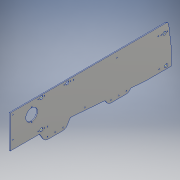
# Autodesk Inventor part: Storage Side Plate
Saved by Autodesk Inventor 2019.4 (Build 234330000, 330)
## iProperties
Created: 2020-01-24
Part Number: Storage Side Plate
Material: Aluminum 6061
Document SubType Name: Modeling
Designer: admin
Density: 2.7 g/cm^3
Appearance: Aluminum - Flat
Mass: 2534.1 g
Surface Area: 3913.12 cm^2
Volume: 938.555 cm^3
Author: admin
Autodesk Inventor part; units mm, degrees
ref_plane "YZ Plane" through (0, 0, 0) normal (1, 0, 0) x (0, 1, 0)
ref_plane "XZ Plane" through (0, 0, 0) normal (0, 1, 0) x (-1, 0, 0)
ref_plane "XY Plane" through (0, 0, 0) normal (0, 0, 1) x (1, 0, 0)
sketch "Sketch1" plane through (0, 0, 0) normal (1, 0, 0) x (0, 1, 0)
  line L0 (0, 0) -> (190, 0)
  line L1 (190, 0) -> (190, -912)
  circle A0 centre (97, -465) radius 88.9 construction
  circle A1 centre (177, -180) radius 9.5
  circle A2 centre (17, -180) radius 9.5
  circle A3 centre (-23, -898.888) radius 9.5
  circle A4 centre (143.8889, -889.1351) radius 9.5
  line L2 (17, -180) -> (-23, -898.888) construction
  line L3 (234.971, -205) -> (-89.3496, -205) construction
  circle A5 centre (175, -330) radius 9.5
  line L4 (175, -330) -> (143.8889, -889.1351) construction
  line L5 (17, -180) -> (177, -180) construction
  circle A6 centre (97, -268.8359) radius 88.9 construction
  circle A7 centre (-93.9984, -625.4651) radius 88.9 construction
  circle A8 centre (-75.5805, -1096.5117) radius 88.9 construction
  circle A9 centre (173.0556, -364.9459) radius 2.75
  circle A10 centre (159.1667, -614.5598) radius 2.75
  circle A11 centre (145.8333, -854.1892) radius 2.75
  circle A12 centre (-20.7778, -858.9498) radius 2.75
  circle A13 centre (-9.1111, -649.2741) radius 2.75
  circle A14 centre (3.1111, -429.6139) radius 2.75
  circle A15 centre (15.0556, -214.9459) radius 2.75
  circle A16 centre (50, -15) radius 2.75
  circle A17 centre (175, -15) radius 2.75
  line L6 (-40, -930) -> (40, -930)
  line L7 (40, -930) -> (190, -912)
  circle A18 centre (-10.6816, -885.7633) radius 2.5 construction
  circle A19 centre (-35.3184, -912.0127) radius 2.5 construction
  line L8 (143.8889, -871.1351) -> (143.8889, -907.1351) construction
  circle A20 centre (143.8889, -871.1351) radius 2.5
  circle A21 centre (143.8889, -907.1351) radius 2.5
  line L9 (17, -162) -> (17, -198) construction
  circle A22 centre (17, -162) radius 2.5
  circle A23 centre (17, -198) radius 2.5
  line L10 (175, -312) -> (175, -348) construction
  circle A24 centre (175, -312) radius 2.5
  circle A25 centre (175, -348) radius 2.5
  line L11 (177, -162) -> (177, -198) construction
  circle A26 centre (177, -162) radius 2.5
  circle A27 centre (177, -198) radius 2.5
  line L12 (-10.6816, -885.7633) -> (-35.3184, -912.0127) construction
  line L13 (0, 0) -> (0, -280)
  line L14 (0, -280) -> (-40, -780)
  line L15 (-40, -780) -> (-40, -930)
  dimension "d1" = 177.8
  dimension "d2" = 19
  dimension "d3" = 19
  dimension "d4" = 19
  dimension "d5" = 19
  dimension "d8" = 180
  dimension "d9" = 180
  dimension "d10" = 205
  dimension "d11" = 19
  dimension "d14" = 125
  dimension "d15" = 190
  dimension "d16" = 18
  dimension "d19" = 160
  dimension "d20" = 560
  dimension "d21" = 720
  dimension "d22" = 177.8
  dimension "d23" = 177.8
  dimension "d24" = 177.8
  dimension "d35" = 5.5
  dimension "d36" = 5.5
  dimension "d37" = 5.5
  dimension "d38" = 35
  dimension "d39" = 35
  dimension "d40" = 250
  dimension "d41" = 5.5
  dimension "d42" = 5.5
  dimension "d43" = 5.5
  dimension "d44" = 5.5
  dimension "d45" = 5.5
  dimension "d46" = 5.5
  dimension "d47" = 35
  dimension "d48" = 40
  dimension "d49" = 250
  dimension "d50" = 250
  dimension "d52" = 15
  dimension "d53" = 15
  dimension "d54" = 15
  dimension "d55" = 80
  dimension "d81" = 5
  dimension "d82" = 5
  dimension "d83" = 36
  dimension "d84" = 5
  dimension "d85" = 5
  dimension "d86" = 36
  dimension "d87" = 5
  dimension "d88" = 5
  dimension "d89" = 36
  dimension "d90" = 5
  dimension "d91" = 5
  dimension "d92" = 36
  dimension "d93" = 5
  dimension "d94" = 5
  dimension "d95" = 36
  dimension "d105" = 930
  dimension "d106" = 40
  dimension "d108" = 50
  dimension "d109" = 500
  dimension "d110" = 17
  dimension "d111" = 17
  dimension "d112" = 40
  dimension "d113" = 150
  dimension "d114" = 15
  constraints: 32 end point, 28 centre point, 10 coincident, 7 point on line, 5 midpoint, 5 vertical, 3 horizontal, 2 parallel, 1 perpendicular
  measures "d1" diameter of A0
  measures "d2" diameter of A1
  measures "d3" diameter of A2
  measures "d4" diameter of A3
  measures "d5" diameter of A4
  measures "d8" distance from line of L5.end L0
  measures "d9" distance from line of L2.start L0
  measures "d10" distance between parallel lines of L0 L3
  measures "d11" diameter of A5
  measures "d14" distance from line of L4.start L3
  measures "d15" distance of L0.start L0.end
  measures "d16" vertical distance of L1.end L6.start
  measures "d19" distance of L2.start L5.end
  measures "d20" distance of L4.end L4.start
  measures "d21" distance of L2.end L2.start
  measures "d22" diameter of A6
  measures "d23" diameter of A7
  measures "d24" diameter of A8
  measures "d35" diameter of A9
  measures "d36" diameter of A10
  measures "d37" diameter of A11
  measures "d38" distance of L4.start A9.centre
  measures "d39" distance of L4.end A11.centre
  measures "d40" distance of A9.centre A10.centre
  measures "d41" diameter of A12
  measures "d42" diameter of A13
  measures "d43" diameter of A14
  measures "d44" diameter of A15
  measures "d45" diameter of A16
  measures "d46" diameter of A17
  measures "d47" distance of L2.start A15.centre
  measures "d48" distance of L2.end A12.centre
  measures "d49" distance of L2.end A13.centre
  measures "d50" distance of L2.start A14.centre
  measures "d52" distance from line of L1 A17.centre
  measures "d53" distance from line of L0 A17.centre
  measures "d54" distance from line of L0 A16.centre
  measures "d55" distance of L6.start L6.end
  measures "d81" diameter of A18
  measures "d82" diameter of A19
  measures "d83" distance of L8.start L8.end
  measures "d84" diameter of A20
  measures "d85" diameter of A21
  measures "d86" distance of L9.start L9.end
  measures "d87" diameter of A22
  measures "d88" diameter of A23
  measures "d89" distance of L10.start L10.end
  measures "d90" diameter of A24
  measures "d91" diameter of A25
  measures "d92" distance of L11.start L11.end
  measures "d93" diameter of A26
  measures "d94" diameter of A27
  measures "d95" distance of L12.start L12.end
  measures "d105" distance between parallel lines of L0 L6
  measures "d106" horizontal distance of L13.end L14.end
  measures "d108" distance from line of L13 A16.centre
  measures "d109" vertical distance of L13.end L14.end
  measures "d110" distance from line of L13 L2.start
  measures "d111" distance from line of L15 L2.end
  measures "d112" angle of L2 L12
  measures "d113" distance of L14.end L6.start
  measures "d114" distance from line of L1 L4.start
extrude "Extrusion1" add sketch "Sketch1" along normal blind 5
ref_plane "Work Plane3" through (5, 1011.7922, 17698.6054) normal (0, -0.9986936, 0.051099) x (-1, 0, 0)
ref_plane "Work Plane1" through (5, 177, -180) normal (0, -0.9989117, 0.0466414) x (-1, 0, 0)
ref_plane "Work Plane2" through (5, -23, -898.888) normal (0, 0.9984556, -0.0555556) x (-1, 0, 0)
ref_plane "Work Plane5" through (5, 177, -245) normal (0, 0, 1) x (-1, 0, 0)
ref_plane "Work Plane4" through (5, 177, -180) normal (0, 0, 1) x (-1, 0, 0)
fillet "Fillet1" radius 15 1 edges at (2.5, 190, -912)
sketch "Sketch2" plane through (5, 0, 0) normal (1, 0, 0) x (0, 0, -1)
  line L0 (780, -40) -> (930, -40) projected
  line L1 (930, -40) -> (865, -40)
  line L2 (865, -40) -> (865, -35)
  line L3 (865, -35) -> (930, -35)
  line L4 (930, -35) -> (930, -40)
  dimension "d115" = 65
  dimension "d116" = 5
  constraints: 8 end point, 2 parallel, 1 horizontal, 1 perpendicular
  measures "d115" distance of L2.end L3.end
  measures "d116" distance of L1.end L2.end
extrude "Extrusion2" [suppressed]
fillet "Fillet3" [suppressed]
sketch "Sketch4" plane through (5, 0, 0) normal (1, 0, 0) x (0, 0, -1)
  circle A0 centre (10, 14.3) radius 2.75 projected
  circle A1 centre (400.3762, 175) radius 2.75 projected
  circle A2 centre (437.8762, 175) radius 2.75 projected
  circle A3 centre (475.3762, 175) radius 2.75 projected
  circle A4 centre (512.8762, 175) radius 2.75 projected
  circle A5 centre (550.3762, 175) radius 2.75 projected
  circle A6 centre (220.7003, 175) radius 2.75 projected
  circle A7 centre (250.7003, 175) radius 2.75 projected
  circle A8 centre (280.7003, 175) radius 2.75 projected
  circle A9 centre (882, -23) radius 2.75 projected
  circle A10 centre (918, -23) radius 2.75 projected
  point P0 (0, 0)
extrude "Extrusion4" [suppressed]
sketch "Sketch5" plane through (5, 0, 0) normal (1, 0, 0) x (0, 0, -1)
  line L0 (865, 0) -> (0, 0) projected
  line L1 (170, 0) -> (200, -50)
  line L2 (200, -50) -> (320, -50)
  line L3 (320, -50) -> (350, 0)
  line L4 (535, 0) -> (565, -50)
  line L5 (565, -50) -> (685, -50)
  line L6 (685, -50) -> (715, 0)
  line L7 (215, -35) -> (305, -35) construction
  circle A0 centre (215, -35) radius 2.75
  circle A1 centre (305, -35) radius 2.75
  circle A2 centre (260, -35) radius 2.75
  line L8 (260, -35) -> (260, -50) construction
  line L9 (580, -35) -> (670, -35) construction
  circle A3 centre (580, -35) radius 2.75
  circle A4 centre (670, -35) radius 2.75
  circle A5 centre (625, -35) radius 2.75
  line L10 (625, -35) -> (625, -50) construction
  dimension "d60" = 30
  dimension "d61" = 120
  dimension "d62" = 120
  dimension "d63" = 30
  dimension "d64" = 50
  dimension "d65" = 200
  dimension "d66" = 180
  dimension "d69" = 5.5
  dimension "d70" = 5.5
  dimension "d71" = 5.5
  dimension "d72" = 90
  dimension "d73" = 15
  dimension "d74" = 5.5
  dimension "d75" = 5.5
  dimension "d76" = 5.5
  dimension "d77" = 90
  dimension "d78" = 15
  constraints: 20 end point, 6 centre point, 6 point on line, 4 coincident, 4 midpoint, 2 equal length, 2 horizontal, 2 perpendicular, 1 parallel
  measures "d60" horizontal distance of L2.end L3.end
  measures "d61" distance of L1.end L2.end
  measures "d62" distance of L4.end L5.end
  measures "d63" horizontal distance of L5.end L6.end
  measures "d64" vertical distance of L1.start L1.end
  measures "d65" horizontal distance of L0.end L1.end
  measures "d66" horizontal distance of L0.start L5.end
  measures "d69" diameter of A0
  measures "d70" diameter of A1
  measures "d71" diameter of A2
  measures "d72" distance of L7.start L7.end
  measures "d73" distance between parallel lines of L2 L7
  measures "d74" diameter of A3
  measures "d75" diameter of A4
  measures "d76" diameter of A5
  measures "d77" distance of L9.start L9.end
  measures "d78" distance of L10.start L10.end
extrude "Extrusion5" add sketch "Sketch5" against normal up to surface (5 mm away)
fillet "Fillet4" radius 30 4 edges at (2.5, -50, -320) (2.5, -50, -200) (2.5, -50, -565) (2.5, -50, -685)
sketch "Sketch6" plane through (5, 0, 0) normal (1, 0, 0) x (0, 0, -1)
  circle A0 centre (123.5866, 120.1489) radius 30.877 construction
  circle A1 centre (123.5866, 120.1489) radius 34
  circle A2 centre (123.5866, 158.6489) radius 2.75
  circle A3 centre (123.5866, 81.6489) radius 2.75
  line L0 (123.5866, 158.6489) -> (123.5866, 81.6489) construction
  point P0 (0, 0)
  dimension "d99" = 68
  dimension "d102" = 5.5
  dimension "d103" = 5.5
  dimension "d104" = 77
  constraints: 4 centre point, 2 coincident, 2 end point, 1 midpoint, 1 vertical, 2 other
  measures "d99" diameter of A1
  measures "d102" diameter of A2
  measures "d103" diameter of A3
  measures "d104" distance of L0.start L0.end
extrude "Extrusion6" cut sketch "Sketch6" against normal through all
body "Solid1"
